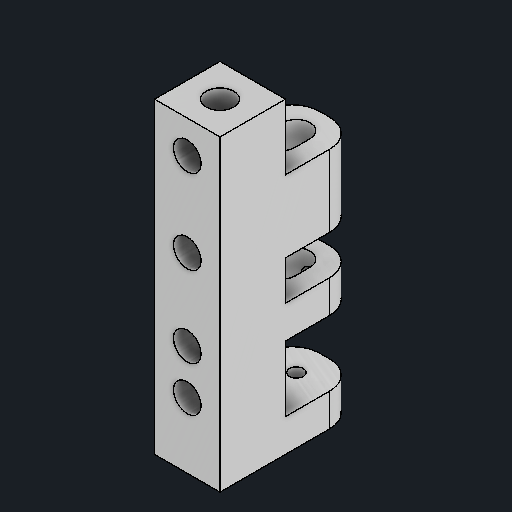
# Autodesk Inventor part: A Idler
Saved by Autodesk Inventor 2026.2 (Build 302298000, 298)
## iProperties
Created: 2025-04-15
Part Number: A Idler
Material: Aluminum 6061
Document SubType Name: Modeling
Designer: Joshua Eah
Density: 2.7 g/cm^3
Appearance: Machined - Aluminum
Author: Joshua Eah
Autodesk Inventor part; units mm, degrees
ref_plane "YZ Plane" through (0, 0, 0) normal (1, 0, 0) x (0, 1, 0)
ref_plane "XZ Plane" through (0, 0, 0) normal (0, 1, 0) x (-1, 0, 0)
ref_plane "XY Plane" through (0, 0, 0) normal (0, 0, 1) x (1, 0, 0)
sketch "Base Profile" plane through (0, 0, 0) normal (0, 1, 0) x (-1, 0, 0)
  line L0 (0, 0) -> (15, 0)
  line L1 (15, 0) -> (15, -15)
  line L2 (15, -15) -> (0, -15)
  line L3 (0, -15) -> (0, 0)
  line L4 (15, 0) -> (31.5, 0)
  line L5 (31.5, 0) -> (31.5, -15)
  line L6 (31.5, -15) -> (15, -15)
  line L7 (15, -15) -> (15, 0)
  line L8 (21.5, -7.5) -> (25, -7.5) construction
  line L9 (21.5, -10.675) -> (25, -10.675)
  line L10 (25, -4.325) -> (21.5, -4.325)
  arc A0 (21.5, -4.325) -> (21.5, -10.675) centre (21.5, -7.5) ccw
  arc A1 (25, -10.675) -> (25, -4.325) centre (25, -7.5) ccw
  point P0 (23.25, -7.5)
  dimension "d164" = 15
  dimension "d165" = 15
  dimension "d166" = 16.5
  dimension "d167" = 15
  dimension "d379" = 6.35
  dimension "d380" = 6.5
  dimension "d381" = 3.5
  dimension "d382" = 7.5
  constraints: 24 end point, 5 parallel, 4 point on circle, 4 tangent, 3 horizontal, 2 centre point, 2 perpendicular, 2 point on line, 1 midpoint
  measures "d164" distance of L1.end L2.end
  measures "d165" distance of L0.end L1.end
  measures "d166" distance of L5.end L6.end
  measures "d167" distance of L4.end L5.end
  measures "d379" diameter of A1
  measures "d380" distance from line of L5 L8.end
  measures "d381" distance of L8.start L8.end
  measures "d382" distance between parallel lines of L4 L8
extrude "Stock" add sketch "Base Profile" along normal blind 70.5 contours L0 L1 L2 L3 | L4 L5 L6 L1 | A0 L10 A1 L9
sketch "Sketch34" plane through (0, 0, -15) normal (0, 0, -1) x (-1, 0, 0)
  line L0 (0, 0) -> (31.5, 0) projected
  line L1 (31.5, 0) -> (31.5, 70.5) projected
  line L2 (0, 70.5) -> (31.5, 70.5) projected
  line L3 (0, 0) -> (0, 70.5) projected
  line L4 (15, 70.5) -> (15, 0)
  line L5 (15, 55.5) -> (31.5, 55.5)
  line L6 (15, 22.5) -> (31.5, 22.5)
  line L7 (15, 7.5) -> (31.5, 7.5)
  line L8 (15, 30) -> (31.5, 30)
  line L9 (15, 39) -> (31.5, 39)
  dimension "d373" = 15
  dimension "d374" = 15
  dimension "d375" = 33
  dimension "d376" = 15
  dimension "d383" = 7.5
  dimension "d384" = 16.5
  constraints: 12 end point, 12 point on line, 5 perpendicular, 1 horizontal
  measures "d373" distance between parallel lines of L4 L3
  measures "d374" distance between parallel lines of L2 L5
  measures "d375" distance between parallel lines of L6 L5
  measures "d376" distance between parallel lines of L7 L6
  measures "d383" distance between parallel lines of L6 L8
  measures "d384" distance between parallel lines of L9 L6
extrude "Extrusion19" cut sketch "Sketch34" against normal through all contours L4 L6 L1 L7 | L2 L1 L5 L4 | L4 L9 L1 L8
extrude "Extrusion20" cut sketch "Base Profile" along normal up to surface (33 mm away) from surface at 22.5 contours A0 L10 A1 L9
sketch "Sketch35" plane through (0, 0, 0) normal (1, 0, 0) x (0, 0, -1)
  line L0 (0, 0) -> (15, 0) projected
  line L1 (15, 0) -> (15, 70.5) projected
  line L2 (0, 70.5) -> (15, 70.5) projected
  line L3 (0, 0) -> (0, 70.5) projected
  circle A0 centre (7.5, 63) radius 3.175
  circle A1 centre (7.5, 43.75) radius 3.175
  circle A2 centre (7.5, 25.25) radius 3.175
  circle A3 centre (7.5, 15) radius 3.175
  line L4 (15, 22.5) -> (0, 22.5) projected
  point P0 (7.5, 70.5)
  dimension "d387" = 6.35
  dimension "d388" = 7.5
  dimension "d389" = 21.25
  dimension "d390" = 2.75
  dimension "d391" = 7.5
  constraints: 4 centre point, 4 vertical alignment, 3 equal radius, 1 midpoint
  measures "d387" diameter of A0
  measures "d388" distance from line of L2 A0.centre
  measures "d389" distance from line of A1.centre L4
  measures "d390" distance from line of L4 A2.centre
  measures "d391" distance from line of A3.centre L4
sketch "Sketch36" plane through (0, 70.5, 0) normal (0, 1, 0) x (1, 0, 0)
  line L0 (-15, 15) -> (-15, 0) projected
  line L1 (-15, 0) -> (0, 0) projected
  line L2 (0, 0) -> (0, 15) projected
  line L3 (0, 15) -> (-15, 15) projected
  circle A0 centre (-7.5, 7.5) radius 3.175
  point P0 (0, 7.5)
  point P1 (-7.5, 0)
  dimension "d392" = 6.35
  constraints: 2 midpoint, 1 centre point, 1 horizontal alignment, 1 vertical alignment
  measures "d392" diameter of A0
hole "Hole24" at (-7.5, 70.5, -7.5) direction (0, -1, 0) diameter 3.2004 end through all counterbore diameter 6.35 counterbore depth 61.674 clearance for "Socket Head Cap Screw" size "M3" standard "Ansi Metric M Profile"
hole "Hole25" at (0, 63, -7.5) at (0, 43.75, -7.5) at (0, 25.25, -7.5) at (0, 15, -7.5) direction (-1, 0, 0) diameter 3.2004 end through all counterbore diameter 6.35 counterbore depth 10.675 clearance for "Socket Head Cap Screw" size "M3" standard "Ansi Metric M Profile"
hole "Hole26" at (-25, 0, -7.5) direction (0, 1, 0) diameter 3.2004 end through all counterbore diameter 6.35 counterbore depth 2.9972 clearance for "Socket Head Cap Screw" size "M3" standard "Ansi Metric M Profile"
fillet "Fillet3" radius 6.35 6 edges at (-31.5, 47.25, 0) (-31.5, 26.25, 0) (-31.5, 3.75, 0) (-31.5, 3.75, -15) (-31.5, 26.25, -15) (-31.5, 47.25, -15)
equation "\"d164\" = extrusionWidth"
equation "\"d165\" = extrusionWidth"
equation "\"d166\" = idlerLength"
equation "\"d167\" = d165"
equation "\"extrusionWidth\" = 15"
equation "\"idlerLength\" = 16.5"
equation "\"bearingOffsetFromBottom\" = 7.5"
equation "\"extrusionOffset\" = 33"
equation "\"bearingStackHeight\" = 9"
equation "\"bearingSlotLength\" = 3.5"
equation "\"bearingClearance\" = 13"
equation "\"pinSupportLength\" = 2"
body "Solid2"
